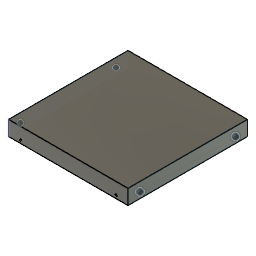
Back Structure (Autodesk Fusion 360 design; units mm, degrees)
part number: 2026-03-10-09-19-59-139
Autodesk Fusion 360 part; units mm, degrees
sketch "Esquisse2" plane through (0, 0, 0) normal (0, 0, 1) x (1, 0, 0)
  line L0 (200, 0) -> (200, 200)
  line L1 (200, 200) -> (0, 200)
  line L2 (0, 200) -> (0, 0)
  line L3 (0, 0) -> (49, 0)
  line L4 (151, 0) -> (200, 0)
  line L5 (49, 0) -> (151, 0)
  dimension "d8" = 200
  dimension "d39" = 102
  constraint vertical L0
  constraint horizontal L1
  constraint vertical L2
  constraint coincident L2.end L3.start
  constraint perpendicular L0 L4
  constraint parallel L4 L5
  measures "d8" distance of L2.end L1.end
  measures "d39" distance of L3.end L4.start
extrude "Extrusion2" add sketch "Esquisse2" along normal blind 25
sketch "Esquisse8" plane through (200, 0, 0) normal (1, 0, 0) x (0, 1, 0)
  line L0 (0, 0) -> (200, 0)
  line L1 (200, 0) -> (200, 25)
  line L2 (200, 25) -> (0, 25)
  line L3 (0, 25) -> (0, 0)
  circle A0 centre (180, 10) radius 2
  circle A1 centre (20, 10) radius 2
  point P0 (180, 10)
  point P1 (20, 10)
  dimension "d40" = 20
  dimension "d41" = 20
  dimension "d42" = 4
  dimension "d43" = 4
  constraint coincident P0 A0.centre
  constraint coincident P1 A1.centre
  measures "d40" distance of L1 P0
  measures "d41" distance of L3 P1
  measures "d42" diameter of A0
  measures "d43" diameter of A1
extrude "Extrusion6" cut sketch "Esquisse8" against normal blind 20 contours A0 | A1
thread "Filetage1" "ISO Metric profile 4.0 M4x0.7 M4x0.7 6H" major diameter 4.1095 minor diameter 3.332 pitch 0.7 angle 60 resizes the face on face at (193.3333, 179.0876, 8.2203) on face at (186.6667, 21.9975, 9.9003)
sketch "Esquisse9" plane through (0, 0, 0) normal (-1, 0, 0) x (0, -1, 0)
  line L0 (-200, 0) -> (0, 0)
  line L1 (0, 25) -> (-200, 25)
  line L2 (-200, 25) -> (-200, 0)
  circle A0 centre (-180, 10) radius 2
  circle A1 centre (-20, 10) radius 2
  line L3 (0, 0) -> (0, 25)
  point P0 (-180, 10)
  point P1 (-20, 10)
  dimension "d49" = 20
  dimension "d50" = 4
  dimension "d51" = 4
  constraint coincident P0 A0.centre
  constraint coincident P1 A1.centre
  measures "d49" distance of L2 P0
  measures "d50" diameter of A0
  measures "d51" diameter of A1
extrude "Extrusion7" cut sketch "Esquisse9" against normal blind 15 contours A0 | A1
thread "Filetage2" "ISO Metric profile 4.0 M4x0.7 M4x0.7 6H" major diameter 4.1095 minor diameter 3.332 pitch 0.7 angle 60 resizes the face on face at (10, 178.6766, 11.4996) on face at (10, 18.0099, 9.8009)
sketch "Esquisse10" plane through (0, 0, 0) normal (0, -1, 0) x (1, 0, 0)
  line L0 (0, 0) -> (49, 0)
  line L1 (49, 0) -> (49, 25)
  line L2 (49, 25) -> (0, 25)
  line L3 (0, 25) -> (0, 0)
  circle A0 centre (20, 5) radius 2
  line L4 (200, 0) -> (200, 25)
  line L5 (0, 25) -> (200, 25)
  circle A1 centre (180, 5) radius 2
  point P0 (20, 5)
  point P1 (180, 5)
  dimension "d56" = 4
  dimension "d57" = 20
  dimension "d58" = 20
  dimension "d59" = 20
  dimension "d60" = 20
  dimension "d61" = 4
  constraint coincident P0 A0.centre
  constraint coincident P1 A1.centre
  measures "d56" diameter of A0
  measures "d57" distance of L3 P0
  measures "d58" distance of L2 P0
  measures "d59" distance of P1 L4
  measures "d60" distance of P1 L5
  measures "d61" diameter of A1
extrude "Extrusion8" cut sketch "Esquisse10" against normal blind 15 contours A0 | A1
thread "Filetage3" "ISO Metric profile 4.0 M4x0.7 M4x0.7 6H" major diameter 4.1095 minor diameter 3.332 pitch 0.7 angle 60 resizes the face on face at (179.0876, 10, 3.2203) on face at (21.9901, 10, 4.8009)
